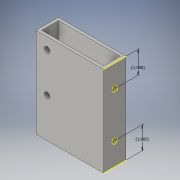
# Autodesk Inventor part: Plate
Saved by Autodesk Inventor 2016 (Build 200138000, 138)
## iProperties
Created: 2016-02-20
Part Number: Plate
Material: Generic
Document SubType Name: Modeling
Designer: Admin
Density: 1 g/cm^3
Appearance: Default
Author: Admin
Autodesk Inventor part; units mm, degrees
ref_plane "YZ Plane" through (0, 0, 0) normal (1, 0, 0) x (0, 1, 0)
ref_plane "XZ Plane" through (0, 0, 0) normal (0, 1, 0) x (-1, 0, 0)
ref_plane "XY Plane" through (0, 0, 0) normal (0, 0, 1) x (1, 0, 0)
sketch "Sketch1" plane through (0, 0, 0) normal (0, 1, 0) x (-1, 0, 0)
  line L0 (0, 0) -> (76.2, 0)
  line L1 (76.2, 0) -> (76.2, 25.4)
  line L2 (76.2, 25.4) -> (0, 25.4)
  line L3 (0, 25.4) -> (0, 0)
  line L4 (73.025, 22.225) -> (73.025, 3.175)
  line L5 (73.025, 3.175) -> (3.175, 3.175)
  line L6 (3.175, 3.175) -> (3.175, 22.225)
  line L7 (3.175, 22.225) -> (73.025, 22.225)
  dimension "d0" = 76.2
  dimension "d1" = 25.4
  dimension "d2" = 3.175
  constraints: 16 end point, 4 parallel, 2 perpendicular, 1 horizontal, 3 other
  measures "d0" distance of L2.end L1.end
  measures "d1" distance of L1.end L0.end
  measures "d2" distance between parallel lines of L1 L4
extrude "Extrusion1" add sketch "Sketch1" along normal blind 101.6
sketch "Sketch2" plane through (0, 0, 25.4) normal (1, 0, 0) x (0, 0, -1)
  circle A0 centre (12.7, 76.2) radius 3.175
  circle A1 centre (12.7, 25.4) radius 3.18
  line L0 (0, 101.6) -> (25.4, 101.6) projected
  line L1 (0, 0) -> (25.4, 0) projected
  dimension "d5" = 6.35
  dimension "d6" = 25.4
  dimension "d7" = 25.4
  constraints: 2 centre point
  measures "d5" diameter of A0
  measures "d6" distance from line of L0 A0.centre
  measures "d7" distance from line of L1 A1.centre
extrude "Extrusion2" cut sketch "Sketch2" against normal blind 3.175
sketch "Sketch3" plane through (-76.2, 0, 25.4) normal (0, 0, 1) x (1, 0, 0)
  circle A0 centre (12.7, 44.45) radius 3.175
  circle A1 centre (12.7, 88.9) radius 3.2003
  line L0 (0, 101.6) -> (76.2, 101.6) projected
  line L1 (0, 0) -> (0, 101.6) projected
  line L2 (0, 0) -> (76.2, 0) projected
  dimension "d10" = 6.35
  dimension "d11" = 12.7
  dimension "d12" = 12.7
  dimension "d13" = 12.7
  dimension "d14" = 44.45
  constraints: 2 centre point
  measures "d10" diameter of A0
  measures "d11" distance from line of L0 A1.centre
  measures "d12" distance from line of L1 A1.centre
  measures "d13" distance from line of L1 A0.centre
  measures "d14" distance from line of L2 A0.centre
extrude "Extrusion3" cut sketch "Sketch3" against normal blind 3.175
sketch "Sketch4" plane through (0, 0, 25.4) normal (1, 0, 0) x (0, 0, -1)
  line L0 (0, 101.6) -> (25.4, 101.6) projected
  circle A0 centre (12.7, 76.2) radius 3.175 projected
  line L1 (0, 0) -> (25.4, 0) projected
  circle A1 centre (12.7, 25.4) radius 3.18 projected
  dimension "d17" = 25.4
  dimension "d18" = 25.4
  measures "d17" distance from line of L0 A0.centre
  measures "d18" distance from line of L1 A1.centre
body "Solid1"
